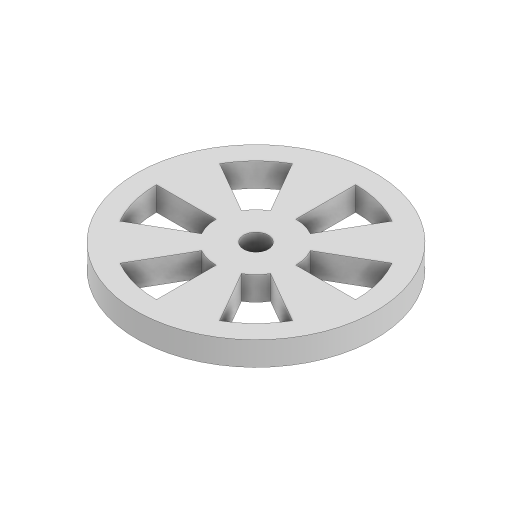
# Autodesk Inventor part: wheel_12_hollow
Saved by Autodesk Inventor 2024 (Build 280153000, 153)
## iProperties
Created: 2024-06-06
Part Number: wheel_12_hollow
Material: 一般
Document SubType Name: Modeling
Designer: USER
Density: 1 g/cm^3
Appearance: 預設
Author: USER
Autodesk Inventor part; units mm, degrees
ref_plane "YZ Plane" through (0, 0, 0) normal (1, 0, 0) x (0, 1, 0)
ref_plane "XZ Plane" through (0, 0, 0) normal (0, 1, 0) x (-1, 0, 0)
ref_plane "XY Plane" through (0, 0, 0) normal (0, 0, 1) x (1, 0, 0)
sketch "草圖1" plane through (0, 0, 0) normal (0, 1, 0) x (-1, 0, 0)
  circle A0 centre (0, 0) radius 15
  line L0 (0, 0) -> (15, 0)
  line L1 (0, 0) -> (7.5, -12.9904)
  line L2 (0, 0) -> (12.9904, -7.5)
  circle A1 centre (0, 0) radius 12.5
  circle A2 centre (0, 0) radius 5
  circle A3 centre (0, 0) radius 1.55
  point P0 (6.25, -10.8253)
  point P1 (2.5, -4.3301)
  point P2 (4.3301, -2.5)
  point P3 (10.8253, -6.25)
  dimension "d0" = 30
  dimension "d1" = 60
  dimension "d2" = 30
  dimension "d3" = 25
  dimension "d4" = 10
  dimension "d12" = 3.1
  constraints: 6 end point, 4 centre point, 4 coincident, 3 point on circle, 1 horizontal
  measures "d0" diameter of A0
  measures "d1" angle of L1 L0
  measures "d2" angle of L0 L2
  measures "d3" diameter of A1
  measures "d4" diameter of A2
  measures "d12" diameter of A3
extrude "擠出1" add sketch "草圖1" along normal blind 3
extrude "擠出2" cut sketch "草圖1" along normal blind 3 contours L1 A2 L2 A1
pattern_circular "環形陣列1" count 6 over 360 about axis through (0, -10, 0) along (0, 1, 0) of "擠出2"
extrude "擠出3" cut sketch "草圖1" along normal blind 3 contours A3 L2 L0 | L0 L1 A3 | L1 L2 A3
